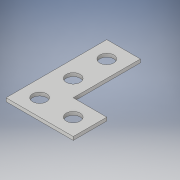
# Autodesk Inventor part: bracing 2x3
Saved by Autodesk Inventor 2018 (Build 220112000, 112)
## iProperties
Created: 2019-01-19
Part Number: bracing 2x3
Material: Generic
Document SubType Name: Modeling
Designer: Burni
Density: 1 g/cm^3
Appearance: Default
Author: Burni
Autodesk Inventor part; units mm, degrees
ref_plane "YZ Plane" through (0, 0, 0) normal (1, 0, 0) x (0, 1, 0)
ref_plane "XZ Plane" through (0, 0, 0) normal (0, 1, 0) x (-1, 0, 0)
ref_plane "XY Plane" through (0, 0, 0) normal (0, 0, 1) x (1, 0, 0)
sketch "Sketch1" plane through (0, 0, 0) normal (0, 1, 0) x (-1, 0, 0)
  line L0 (0, 0) -> (-25.4, 0)
  line L1 (-25.4, 0) -> (-25.4, 76.2)
  line L2 (-25.4, 76.2) -> (0, 76.2)
  line L3 (0, 76.2) -> (0, 0)
  line L4 (-25.4, 76.2) -> (-50.8, 76.2)
  line L5 (-50.8, 76.2) -> (-50.8, 50.8)
  line L6 (-50.8, 50.8) -> (-25.4, 50.8)
  line L7 (-25.4, 50.8) -> (-25.4, 76.2)
  circle A0 centre (-12.7, 12.7) radius 5.2917
  circle A1 centre (-38.1, 63.5) radius 5.2917
  circle A2 centre (-12.7, 38.1) radius 5.2917
  circle A3 centre (-12.7, 63.5) radius 5.2917
  dimension "d0" = 76.2
  dimension "d1" = 25.4
  dimension "d2" = 25.4
  dimension "d3" = 25.4
  dimension "d5" = 38.1
  dimension "d7" = 25.4
  dimension "d8" = 25.4
  dimension "d11" = 12.7
  dimension "d12" = 12.7
  dimension "d13" = 12.7
  dimension "d14" = 10.5833
  dimension "d15" = 10.5833
  dimension "d16" = 10.5833
  dimension "d17" = 10.5833
  dimension "d18" = 12.7
  dimension "d19" = 25.4
  dimension "d20" = 12.7
  constraints: 16 end point, 4 centre point, 4 parallel, 2 horizontal, 2 perpendicular
  measures "d0" distance of L0.end L1.end
  measures "d1" distance of L1.end L2.end
  measures "d2" distance of L1.end L4.end
  measures "d3" distance of L4.end L5.end
  measures "d5" distance from line of L5 A3.centre
  measures "d7" horizontal distance of A1.centre A2.centre
  measures "d8" distance of A2.centre A0.centre
  measures "d11" distance from line of L3 A2.centre
  measures "d12" distance from line of L0 A0.centre
  measures "d13" distance from line of L2 A1.centre
  measures "d14" diameter of A0
  measures "d15" diameter of A2
  measures "d16" diameter of A1
  measures "d17" diameter of A3
  measures "d18" distance from line of L5 A1.centre
  measures "d19" distance of A1.centre A3.centre
  measures "d20" distance from line of L2 A3.centre
extrude "Extrusion1" add sketch "Sketch1" along normal blind 2.54
equation "\"d15\" = d14"
equation "\"d16\" = d14"
equation "\"d17\" = d14"
body "Solid1"
